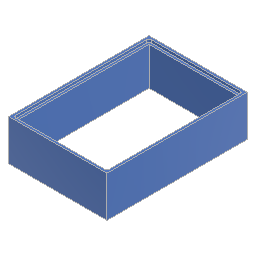
Binder-Clamps-Holder (Autodesk Fusion 360 design; units mm, degrees)
Autodesk Fusion 360 part; units mm, degrees
sketch "Sketch3" plane through (0, 0, 3.175) normal (0, 0, 1) x (-1, 0, 0)
  line L0 (0, 0) -> (0, 297.942)
  line L1 (0, 297.942) -> (-407.924, 297.942)
  line L2 (-407.924, 297.942) -> (-407.924, 0)
  line L3 (-407.924, 0) -> (0, 0)
sketch "Sketch1" plane through (0, 0, 3.175) normal (0, 0, 1) x (-1, 0, 0)
  line L0 (0, 0) -> (0, 297.942)
  line L1 (0, 297.942) -> (-407.924, 297.942)
  line L2 (-407.924, 297.942) -> (-407.924, 0)
  line L3 (-407.924, 0) -> (0, 0)
  line L4 (-201.1, 236.942) -> (-201.1, 297.942)
  line L5 (-319.424, 180) -> (-407.924, 180)
  line L6 (-201.1, 297.942) -> (-285.1, 297.942)
  line L7 (-285.1, 297.942) -> (-285.1, 177.942)
  line L8 (-285.1, 177.942) -> (-201.1, 177.942)
  line L9 (-201.1, 177.942) -> (-201.1, 297.942)
  line L10 (-205.1, 293.942) -> (-281.1, 293.942)
  line L11 (-281.1, 293.942) -> (-281.1, 181.942)
  line L12 (-281.1, 181.942) -> (-205.1, 181.942)
  line L13 (-205.1, 181.942) -> (-205.1, 293.942)
  dimension "d153" = 120
  dimension "d154" = 84
  constraint horizontal L6
  constraint vertical L7
  constraint horizontal L8
  constraint vertical L9
  constraint coincident L4.end L6.start
  measures "d153" distance of L6.end L7.end
  measures "d154" distance of L4.end L6.end
extrude "Extrude1" add sketch "Sketch1" along normal blind 35 contours L1 L4 L6 L7 L8 L9
sketch "Sketch2" plane through (0, 0, 38.175) normal (0, 0, 1) x (-1, 0, 0)
  line L0 (-205.1, 293.942) -> (-205.1, 181.942)
  line L1 (-205.1, 181.942) -> (-281.1, 181.942)
  line L2 (-281.1, 181.942) -> (-281.1, 293.942)
  line L3 (-281.1, 293.942) -> (-205.1, 293.942)
  line L4 (-201.1, 177.942) -> (-201.1, 297.942)
  line L5 (-201.1, 297.942) -> (-285.1, 297.942)
  line L6 (-285.1, 297.942) -> (-285.1, 177.942)
  line L7 (-285.1, 177.942) -> (-201.1, 177.942)
  line L8 (-205.1, 293.942) -> (-205.1, 181.942)
  line L9 (-205.1, 181.942) -> (-281.1, 181.942)
  line L10 (-281.1, 181.942) -> (-281.1, 293.942)
  line L11 (-281.1, 293.942) -> (-205.1, 293.942)
  line L12 (-205.1, 179.942) -> (-281.1, 179.942)
  line L13 (-283.1, 181.942) -> (-283.1, 293.942)
  line L14 (-281.1, 295.942) -> (-205.1, 295.942)
  line L15 (-203.1, 293.942) -> (-203.1, 181.942)
  arc A0 (-281.1, 295.942) -> (-283.1, 293.942) centre (-281.1, 293.942) ccw
  arc A1 (-283.1, 181.942) -> (-281.1, 179.942) centre (-281.1, 181.942) ccw
  arc A2 (-205.1, 179.942) -> (-203.1, 181.942) centre (-205.1, 181.942) ccw
  arc A3 (-203.1, 293.942) -> (-205.1, 295.942) centre (-205.1, 293.942) ccw
  dimension "d159" = 2
  constraint tangent L14 A0
  constraint tangent L13 A0
  constraint tangent L13 A1
  constraint tangent L12 A1
  constraint equal A0 A1
  constraint tangent L12 A2
  constraint tangent L15 A2
  constraint equal A0 A2
  constraint tangent L15 A3
  constraint tangent L14 A3
  constraint equal A0 A3
  measures "d159" radius of A0
extrude "Extrude2" cut sketch "Sketch2" against normal blind 2.5 contours L0 L1 L2 L3 L8 L9 L10 L11 | L12 L13 L14 L15 A0 A1 A2 A3
equation "d153 = 118 mm + ( ComponentWallWidth / 2 )"
equation "d154 = 82 mm + ( ComponentWallWidth / 2 )"
equation "d155 = -ComponentWallWidth"
equation "ComponentWallWidth = 4 mm"
